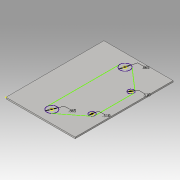
# Autodesk Inventor part: recreated v of plate
Saved by Autodesk Inventor 2016 (Build 200138000, 138)
## iProperties
Created: 2015-11-23
Part Number: recreated v of plate
Material: Generic
Document SubType Name: Modeling
Designer: Delta
Density: 1 g/cm^3
Appearance: Default
Author: Delta
Autodesk Inventor part; units mm, degrees
ref_plane "YZ Plane" through (0, 0, 0) normal (1, 0, 0) x (0, 1, 0)
ref_plane "XZ Plane" through (0, 0, 0) normal (0, 1, 0) x (-1, 0, 0)
ref_plane "XY Plane" through (0, 0, 0) normal (0, 0, 1) x (1, 0, 0)
sketch "Sketch3" plane through (0, 0, 0) normal (0, 1, 0) x (-1, 0, 0)
  line L0 (0, 0) -> (-152.4, 0)
  line L1 (-152.4, 0) -> (-152.4, -215.9)
  line L2 (-152.4, -215.9) -> (0, -215.9)
  line L3 (0, -215.9) -> (0, 0)
  dimension "d8" = 152.4
  dimension "d9" = 215.9
  constraints: 8 end point, 2 parallel, 1 horizontal, 1 perpendicular
  measures "d8" distance of L2.end L1.end
  measures "d9" distance of L1.end L0.end
extrude "Extrusion1" add sketch "Sketch3" against normal blind 3.175
sketch "Sketch4" plane through (0, 0, 0) normal (0, 1, 0) x (1, 0, 0)
  line L0 (152.4, 0) -> (152.4, 215.9) projected
  line L1 (0, 0) -> (152.4, 0) projected
  line L2 (152.4, 215.9) -> (0, 215.9) projected
  point P0 (126.3904, 63.0378)
  point P1 (126.3904, 148.7849)
  point P2 (73.406, 188.5442)
  point P3 (73.406, 27.3558)
  dimension "d12" = 26.0096
  dimension "d13" = 26.0096
  dimension "d14" = 78.994
  dimension "d15" = 78.994
  dimension "d16" = 27.3558
  dimension "d17" = 27.3558
  dimension "d29" = 63.0378
  dimension "d30" = 67.1151
  measures "d12" distance from line of L0 point (126.39, 63.038)
  measures "d13" distance from line of L0 point (126.39, 148.785)
  measures "d14" distance from line of L0 point (73.406, 188.544)
  measures "d15" distance from line of L0 point (73.406, 27.356)
  measures "d16" distance from line of point (73.406, 27.356) L1
  measures "d17" distance from line of L2 point (73.406, 188.544)
  measures "d29" distance from line of point (126.39, 63.038) L1
  measures "d30" distance from line of L2 point (126.39, 148.785)
hole "Hole1" at (126.3904, 0, -63.0378) at (126.3904, 0, -148.7849) at (73.406, 0, -188.5442) at (73.406, 0, -27.3558) direction (0, -1, 0) diameter 5.9944 end through all
sketch "Sketch5" plane through (0, 0, 0) normal (0, 1, 0) x (1, 0, 0)
  circle A0 centre (126.3904, 148.7849) radius 2.9972 projected
  circle A1 centre (126.3904, 148.7849) radius 6.477
  circle A2 centre (126.3904, 63.0378) radius 2.9972 projected
  circle A3 centre (126.3904, 63.0378) radius 6.477
  circle A4 centre (73.406, 27.3558) radius 2.9972 projected
  circle A5 centre (73.406, 27.3558) radius 10.9855
  circle A6 centre (73.406, 188.5442) radius 2.9972 projected
  circle A7 centre (73.406, 188.5442) radius 10.9855
  line L0 (131.1992, 58.6988) -> (80.1831, 18.7099)
  line L1 (132.8674, 63.0378) -> (132.8674, 148.7849)
  line L2 (80.1831, 197.1901) -> (129.3876, 154.5267)
  line L3 (62.4205, 27.3558) -> (62.4205, 188.5442)
  point P0 (0, 0)
  dimension "d25" = 12.954
  dimension "d26" = 12.954
  dimension "d27" = 21.971
  dimension "d28" = 21.971
  constraints: 8 end point, 8 point on circle, 4 centre point, 4 coincident, 2 tangent, 1 vertical
  measures "d25" diameter of A1
  measures "d26" diameter of A3
  measures "d27" diameter of A5
  measures "d28" diameter of A7
equation "\"d13\" = d12"
equation "\"d15\" = d14"
equation "\"d17\" = d16"
body "Solid1"
